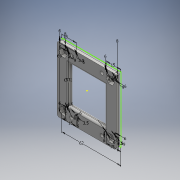
# Autodesk Inventor part: BatteryHolder2PBase
Saved by Autodesk Inventor 2016 (Build 200138000, 138)
## iProperties
Created: 2026-05-01
Part Number: BatteryHolder2PBase
Material: Generic
Document SubType Name: Modeling
Designer: Steve
Density: 1 g/cm^3
Appearance: Default
Author: Steve
Autodesk Inventor part; units mm, degrees
ref_plane "YZ Plane" through (0, 0, 0) normal (1, 0, 0) x (0, 1, 0)
ref_plane "XZ Plane" through (0, 0, 0) normal (0, 1, 0) x (-1, 0, 0)
ref_plane "XY Plane" through (0, 0, 0) normal (0, 0, 1) x (1, 0, 0)
sketch "Sketch1" plane through (0, 0, 0) normal (0, 1, 0) x (-1, 0, 0)
  line L0 (26.2836, 34.9539) -> (-35.7164, 34.9539)
  line L1 (-35.7164, 34.9539) -> (-35.7164, -34.0461)
  line L2 (-35.7164, -34.0461) -> (26.2836, -34.0461)
  line L3 (26.2836, -34.0461) -> (26.2836, 34.9539)
  circle A0 centre (11.2836, -28.0461) radius 1.75
  circle A1 centre (11.2836, -28.0461) radius 3
  circle A2 centre (-20.7164, -28.0461) radius 1.75
  circle A3 centre (-20.7164, -28.0461) radius 3
  circle A4 centre (-20.7164, 28.9539) radius 1.75
  circle A5 centre (-20.7164, 28.9539) radius 3
  circle A6 centre (11.2836, 28.9539) radius 1.75
  circle A7 centre (11.2836, 28.9539) radius 3
  line L4 (-15.7164, 34.9539) -> (-25.7164, 34.9539)
  circle A8 centre (20.2836, 26.9539) radius 2.25
  circle A9 centre (20.2836, -26.0461) radius 2.25
  circle A10 centre (-29.7164, 26.9539) radius 2.25
  circle A11 centre (-29.7164, -26.0461) radius 2.25
  circle A12 centre (20.2836, 26.9539) radius 4.5
  circle A13 centre (20.2836, -26.0461) radius 4.5
  circle A14 centre (-29.7164, -26.0461) radius 4.5
  circle A15 centre (-29.7164, 26.9539) radius 4.5
  line L5 (18.0336, 23.0568) -> (15.7836, 26.9539)
  line L6 (15.7836, 26.9539) -> (18.0336, 30.8511)
  line L7 (18.0336, 30.8511) -> (22.5336, 30.8511)
  line L8 (22.5336, 30.8511) -> (24.7836, 26.9539)
  line L9 (24.7836, 26.9539) -> (22.5336, 23.0568)
  line L10 (22.5336, 23.0568) -> (18.0336, 23.0568)
  line L11 (18.0336, -29.9432) -> (15.7836, -26.0461)
  line L12 (15.7836, -26.0461) -> (18.0336, -22.1489)
  line L13 (18.0336, -22.1489) -> (22.5336, -22.1489)
  line L14 (22.5336, -22.1489) -> (24.7836, -26.0461)
  line L15 (24.7836, -26.0461) -> (22.5336, -29.9432)
  line L16 (22.5336, -29.9432) -> (18.0336, -29.9432)
  line L17 (-31.9664, -29.9432) -> (-34.2164, -26.0461)
  line L18 (-34.2164, -26.0461) -> (-31.9664, -22.1489)
  line L19 (-31.9664, -22.1489) -> (-27.4664, -22.1489)
  line L20 (-27.4664, -22.1489) -> (-25.2164, -26.0461)
  line L21 (-25.2164, -26.0461) -> (-27.4664, -29.9432)
  line L22 (-27.4664, -29.9432) -> (-31.9664, -29.9432)
  line L23 (-31.9664, 23.0568) -> (-34.2164, 26.9539)
  line L24 (-34.2164, 26.9539) -> (-31.9664, 30.8511)
  line L25 (-31.9664, 30.8511) -> (-27.4664, 30.8511)
  line L26 (-27.4664, 30.8511) -> (-25.2164, 26.9539)
  line L27 (-25.2164, 26.9539) -> (-27.4664, 23.0568)
  line L28 (-27.4664, 23.0568) -> (-31.9664, 23.0568)
  point P0 (0, 0)
  dimension "d45" = 9
  dimension "d46" = 9
  dimension "d47" = 9
  dimension "d48" = 9
  dimension "d0" = 69
  dimension "d1" = 62
  dimension "d2" = 3.5
  dimension "d3" = 6
  dimension "d4" = 3.5
  dimension "d5" = 6
  dimension "d6" = 3.5
  dimension "d7" = 6
  dimension "d8" = 3.5
  dimension "d9" = 6
  dimension "d10" = 15
  dimension "d11" = 15
  dimension "d12" = 15
  dimension "d13" = 15
  dimension "d14" = 6
  dimension "d15" = 6
  dimension "d16" = 6
  dimension "d17" = 6
  dimension "d32" = 4.5
  dimension "d33" = 4.5
  dimension "d34" = 4.5
  dimension "d35" = 4.5
  dimension "d36" = 8
  dimension "d37" = 8
  dimension "d38" = 8
  dimension "d39" = 8
  dimension "d40" = 6
  dimension "d41" = 6
  dimension "d42" = 6
  dimension "d43" = 6
  dimension "d44" = 53
  constraints: 58 end point, 12 centre point, 12 coincident, 3 point on line, 2 horizontal, 2 parallel, 1 perpendicular, 64 other
  measures "d0" distance of L2.end L0.start
  measures "d1" distance of L1.end L2.end
  measures "d2" diameter of A0
  measures "d3" diameter of A1
  measures "d4" diameter of A2
  measures "d5" diameter of A3
  measures "d6" diameter of A4
  measures "d7" diameter of A5
  measures "d8" diameter of A6
  measures "d9" diameter of A7
  measures "d10" distance from line of L3 A0.centre
  measures "d11" distance from line of L1 A3.centre
  measures "d12" distance from line of L1 A4.centre
  measures "d13" distance from line of L3 A6.centre
  measures "d14" distance from line of L2 A0.centre
  measures "d15" distance from line of L2 A2.centre
  measures "d16" distance from line of L0 A4.centre
  measures "d17" distance from line of L0 A6.centre
  measures "d32" diameter of A8
  measures "d33" diameter of A9
  measures "d34" diameter of A10
  measures "d35" diameter of A11
  measures "d36" distance from line of L0 A8.centre
  measures "d37" distance from line of L2 A9.centre
  measures "d38" distance from line of L2 A11.centre
  measures "d39" distance from line of L0 A10.centre
  measures "d40" distance from line of L1 A10.centre
  measures "d41" distance from line of L1 A11.centre
  measures "d42" distance from line of L3 A9.centre
  measures "d43" distance from line of L3 A8.centre
  measures "d44" distance of A9.centre A8.centre
extrude "Extrusion1" add sketch "Sketch1" against normal blind 5 contours L3 L2 L1 L0 | A1 | A3 | A5 | A7 | L8 A12 | L9 L10 L5 L6 L7 L8 | A12 L9 | L7 A12 | A12 L10 | L6 A12 | A12 L5 | L14 A13 | L15 L16 L11 L12 L13 L14 | A13 L15 | L13 A13 | A13 L16 | L12 A13 | A13 L11 | L20 A14 | L21 L22 L17 L18 L19 L20 | A14 L21 | L19 A14 | A14 L22 | L18 A14 | A14 L17 | L26 A15 | L27 L28 L23 L24 L25 L26 | A15 L27 | L25 A15 | A15 L28 | L24 A15 | A15 L23
extrude "Extrusion2" cut sketch "Sketch1" against normal blind 2 contours A1 | A3 | A5 | A7
sketch "Sketch2" plane through (0, -5, 0) normal (0, -1, 0) x (1, 0, 0)
  line L0 (27.5264, 23.0228) -> (25.2764, 26.92)
  line L1 (25.2764, 26.92) -> (27.5264, 30.8171)
  line L2 (27.5264, 30.8171) -> (32.0264, 30.8171)
  line L3 (32.0264, 30.8171) -> (34.279, 26.9154)
  line L4 (34.279, 26.9154) -> (32.0264, 23.0198)
  line L5 (32.0264, 23.0198) -> (27.5264, 23.0228)
  line L6 (27.4664, -29.9432) -> (25.2764, -26.0461)
  line L7 (25.2764, -26.0461) -> (27.5264, -22.1489)
  line L8 (27.5264, -22.1489) -> (32.0264, -22.1489)
  line L9 (32.0264, -22.1489) -> (34.2164, -26.0461)
  line L10 (34.2164, -26.0461) -> (31.9664, -29.9432)
  line L11 (31.9664, -29.9432) -> (27.4664, -29.9432)
  line L12 (-22.5336, -29.9432) -> (-24.7836, -26.0461)
  line L13 (-24.7836, -26.0461) -> (-22.5336, -22.1489)
  line L14 (-22.5336, -22.1489) -> (-18.0336, -22.1489)
  line L15 (-18.0336, -22.1489) -> (-15.7836, -26.0461)
  line L16 (-15.7836, -26.0461) -> (-18.0336, -29.9432)
  line L17 (-18.0336, -29.9432) -> (-22.5336, -29.9432)
  line L18 (-22.5336, 23.0568) -> (-24.7236, 26.9539)
  line L19 (-24.7236, 26.9539) -> (-22.4736, 30.8511)
  line L20 (-22.4736, 30.8511) -> (-17.9736, 30.8511)
  line L21 (-17.9736, 30.8511) -> (-15.7236, 26.9539)
  line L22 (-15.7236, 26.9539) -> (-17.9736, 23.0568)
  line L23 (-17.9736, 23.0568) -> (-22.5336, 23.0568)
  line L24 (-26.2836, 34.9539) -> (-26.2836, -34.0461) projected
  line L25 (35.7164, 34.9539) -> (-26.2836, 34.9539) projected
  line L26 (35.7164, -34.0461) -> (35.7164, 34.9539) projected
  line L27 (-26.2836, -34.0461) -> (35.7164, -34.0461) projected
  point P0 (0, 0)
  constraints: 48 end point, 2 point on line
extrude "Extrusion3" cut sketch "Sketch2" against normal blind 4 contours L0 L1 L2 L3 L4 L5 | L6 L7 L8 L9 L10 L11 | L12 L13 L14 L15 L16 L17 | L18 L19 L20 L21 L22 L23
fillet "Fillet1" radius 2 8 edges at (35.7164, -2.5, -34.0461) (35.7164, -2.5, 34.9539) (-26.2836, -2.5, 34.9539) (-26.2836, -2.5, -34.0461) (-26.2836, 0, 0.4539) (4.7164, 0, -34.0461) (4.7164, 0, 34.9539) (35.7164, 0, 0.4539)
sketch "Sketch3" plane through (0, 0, 0) normal (0, 1, 0) x (1, 0, 0)
  line L0 (23.7164, 19.0461) -> (-14.2836, 19.0461)
  line L1 (-14.2836, 19.0461) -> (-14.2836, -19.9539)
  line L2 (-14.2836, -19.9539) -> (23.7164, -19.9539)
  line L3 (23.7164, -19.9539) -> (23.7164, 19.0461)
  line L4 (35.7164, -32.9539) -> (35.7164, 32.0461) projected
  line L5 (-26.2836, 32.0461) -> (-26.2836, -32.9539) projected
  line L6 (-24.2836, -34.9539) -> (33.7164, -34.9539) projected
  line L7 (33.7164, 34.0461) -> (-24.2836, 34.0461) projected
  point P0 (0, 0)
  dimension "d68" = 12
  dimension "d69" = 12
  dimension "d70" = 15
  dimension "d71" = 15
  constraints: 8 end point, 2 parallel, 1 horizontal, 1 perpendicular
  measures "d68" distance between parallel lines of L4 L3
  measures "d69" distance between parallel lines of L5 L1
  measures "d70" distance between parallel lines of L6 L2
  measures "d71" distance between parallel lines of L7 L0
extrude "Extrusion4" cut sketch "Sketch3" against normal through all
fillet "Fillet2" radius 2 8 edges at (4.7164, 0, -19.0461) (23.7164, 0, 0.4539) (4.7164, 0, 19.9539) (-14.2836, 0, 0.4539) (4.7164, -5, 19.9539) (-14.2836, -5, 0.4539) (4.7164, -5, -19.0461) (23.7164, -5, 0.4539)
body "Solid1"
